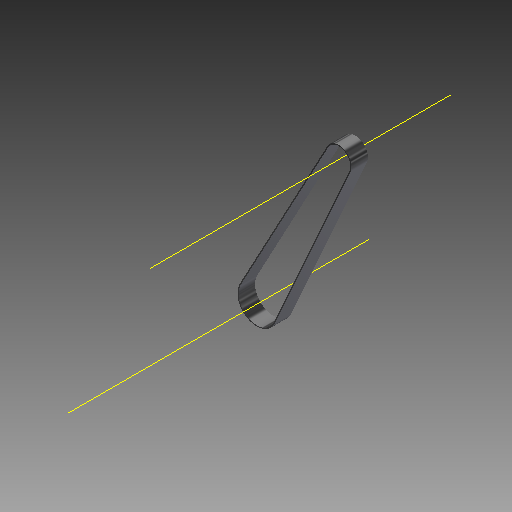
# Autodesk Inventor part: Synchronous Belt
Saved by Autodesk Inventor 2019.4 (Build 234330000, 330)
## iProperties
Created: 2020-01-18
Part Number: Synchronous Belt
Material: Rubber
Document SubType Name: Modeling
Designer: admin
Density: 1 g/cm^3
Appearance: Rubber - Black - Version 1.1
CustomPartVersion: 1
Author: admin
Autodesk Inventor part; units mm, degrees
ref_plane "YZ Plane" through (0, 0, 0) normal (1, 0, 0) x (0, 1, 0)
ref_plane "XZ Plane" through (0, 0, 0) normal (0, 1, 0) x (-1, 0, 0)
ref_plane "XY Plane" through (0, 0, 0) normal (0, 0, 1) x (1, 0, 0)
sketch "Sketch Path" plane through (0, 0, 0) normal (0, 0, 1) x (1, 0, 0)
  arc A0 (-177.7963, -54.5344) -> (-144.9775, -70.6968) centre (-161.6731, -63.1967) ccw
  arc A1 (-71.3095, 93.2904) -> (-92.713, 103.8312) centre (-82.1979, 98.1818) ccw
  line L0 (-71.3095, 93.2904) -> (-144.9775, -70.6968)
  line L1 (-177.7963, -54.5344) -> (-92.713, 103.8312)
  constraints: 4 end point, 4 point on circle, 2 centre point
ref_plane "Cross Section Plane" through (-144.9775, -70.6968, 0) normal (0.4097804, 0.9121842, 0) x (0, 0, 1)
ref_plane "Work Plane2" through (-161.6731, -63.1967, 0) normal (-1, 0, 0) x (0, 0, 1)
ref_plane "Work Plane3" through (-82.1979, 98.1818, 0) normal (-0.7882049, -0.6154129, 0) x (0, 0, 1)
sketch "Cross Section" plane through (-144.9775, -70.6968, 0) normal (0.4097804, 0.9121842, 0) x (0, 0, 1)
  line L0 (-8, 0.5) -> (8, 0.5)
  line L1 (8, 0.5) -> (8, -0.5)
  line L2 (8, -0.5) -> (-8, -0.5)
  line L3 (-8, -0.5) -> (-8, 0.5)
  line L4 (-8, 0) -> (8, 0) construction
  point P0 (0, 0)
  point P1 (0, 0)
  dimension "d0" = 16
  dimension "d4" = 0.5
  dimension "d5" = 0.5
  constraints: 10 end point, 3 midpoint, 2 parallel, 1 coincident, 1 horizontal, 1 perpendicular, 1 other
  measures "d0" distance between parallel lines of L1 L3
  measures "d4" distance between parallel lines of L2 L4
  measures "d5" distance between parallel lines of L4 L0
sweep "Belt" add profiles "Cross Section" path "Sketch Path" path curves L1 A1 L0 A0
equation "\"d0\" = da_B"
equation "\"d4\" = da_a"
equation "\"d5\" = da_a2"
equation "\"da_B\" = 16"
equation "\"da_pb\" = 5"
equation "\"da_L\" = 454.99932"
equation "\"da_a\" = 0.5"
equation "\"da_S\" = 2.65"
equation "\"da_Beta\" = 20deg"
equation "\"da_Ht\" = 1.2"
equation "\"da_H\" = 2.2"
equation "\"da_a2\" = 0.5"
body "Solid1"
